Autodesk Fusion 360 part; units mm, degrees
(part 18 of 25)
  arc A5071 (10.428, 31.5912) -> (10.428, 31.9088) centre (10.428, 31.75) ccw
  arc A5072 (0.7747, 31.9088) -> (0.7747, 31.5912) centre (0.7747, 31.75) ccw
  arc A5073 (84.2253, 30.3212) -> (84.2253, 30.6388) centre (84.2253, 30.48) ccw
  arc A5074 (9.3135, 30.6388) -> (9.3135, 30.3212) centre (9.3135, 30.48) ccw
  arc A5075 (81.28, 31.2738) -> (81.28, 30.9563) centre (81.28, 31.1151) ccw
  arc A5076 (12.5375, 32.8613) -> (12.5375, 33.1788) centre (12.5375, 33.0201) ccw
  arc A5077 (0.7747, 31.2738) -> (0.7747, 30.9563) centre (0.7747, 31.1151) ccw
  arc A5078 (26.9586, 30.9563) -> (26.9586, 31.2738) centre (26.9586, 31.1151) ccw
  arc A5079 (84.2253, 29.6863) -> (84.2253, 30.0038) centre (84.2253, 29.8451) ccw
  arc A5080 (17.7173, 31.9088) -> (17.7173, 31.5912) centre (17.7173, 31.75) ccw
  arc A5081 (37.7536, 31.5912) -> (37.7536, 31.9088) centre (37.7536, 31.75) ccw
  arc A5082 (71.8947, 30.9563) -> (71.8947, 31.2738) centre (71.8947, 31.1151) ccw
  arc A5083 (66.04, 30.0038) -> (66.04, 29.6863) centre (66.04, 29.8451) ccw
  arc A5084 (67.5178, 30.6388) -> (67.5178, 30.3212) centre (67.5178, 30.48) ccw
  arc A5085 (66.04, 30.6388) -> (66.04, 30.3212) centre (66.04, 30.48) ccw
  arc A5086 (50.5114, 31.2738) -> (50.5114, 30.9563) centre (50.5114, 31.1151) ccw
  arc A5087 (49.9686, 31.5912) -> (49.9686, 31.9088) centre (49.9686, 31.75) ccw
  arc A5088 (47.9714, 33.8137) -> (47.9714, 33.4963) centre (47.9714, 33.655) ccw
  arc A5089 (1.0423, 33.4963) -> (1.0423, 33.8137) centre (1.0423, 33.655) ccw
  arc A5090 (71.8947, 32.2263) -> (71.8947, 32.5437) centre (71.8947, 32.385) ccw
  arc A5091 (67.5513, 32.5437) -> (67.5513, 32.2263) centre (67.5513, 32.385) ccw
  arc A5092 (59.1947, 32.2263) -> (59.1947, 32.5437) centre (59.1947, 32.385) ccw
  arc A5093 (4.5252, 33.1788) -> (4.5252, 32.8613) centre (4.5252, 33.0201) ccw
  arc A5094 (59.1947, 32.8613) -> (59.1947, 33.1788) centre (59.1947, 33.0201) ccw
  arc A5095 (54.786, 33.4963) -> (54.786, 33.8137) centre (54.786, 33.655) ccw
  arc A5096 (13.194, 31.9088) -> (13.194, 31.5912) centre (13.194, 31.75) ccw
  arc A5097 (56.974, 33.8137) -> (56.974, 33.4963) centre (56.974, 33.655) ccw
  arc A5098 (81.28, 32.2263) -> (81.28, 32.5437) centre (81.28, 32.385) ccw
  arc A5099 (0.7747, 33.1788) -> (0.7747, 32.8613) centre (0.7747, 33.0201) ccw
  arc A5100 (49.3336, 32.2263) -> (49.3336, 32.5437) centre (49.3336, 32.385) ccw
  arc A5101 (15.127, 31.5912) -> (15.127, 31.9088) centre (15.127, 31.75) ccw
  arc A5102 (66.04, 33.8137) -> (66.04, 33.4963) centre (66.04, 33.655) ccw
  arc A5103 (59.4491, 33.4963) -> (59.4491, 33.8137) centre (59.4491, 33.655) ccw
  arc A5104 (67.5178, 33.1788) -> (67.5178, 32.8613) centre (67.5178, 33.0201) ccw
  arc A5105 (67.2068, 33.8137) -> (67.2068, 33.4963) centre (67.2068, 33.655) ccw
  arc A5106 (72.1491, 33.4963) -> (72.1491, 33.8137) centre (72.1491, 33.655) ccw
  arc A5107 (49.2414, 32.5437) -> (49.2414, 32.2263) centre (49.2414, 32.385) ccw
  arc A5108 (1.5708, 32.8613) -> (1.5708, 33.1788) centre (1.5708, 33.0201) ccw
  arc A5109 (66.04, 32.2263) -> (66.04, 32.5437) centre (66.04, 32.385) ccw
  arc A5110 (12.559, 32.5437) -> (12.559, 32.2263) centre (12.559, 32.385) ccw
  arc A5111 (9.793, 32.2263) -> (9.793, 32.5437) centre (9.793, 32.385) ccw
  arc A5112 (81.28, 33.4963) -> (81.28, 33.8137) centre (81.28, 33.655) ccw
  arc A5113 (17.7419, 32.5437) -> (17.7419, 32.2263) centre (17.7419, 32.385) ccw
  arc A5114 (15.762, 32.2263) -> (15.762, 32.5437) centre (15.762, 32.385) ccw
  arc A5115 (66.04, 32.5437) -> (66.04, 32.2263) centre (66.04, 32.385) ccw
  arc A5116 (6.6508, 32.8613) -> (6.6508, 33.1788) centre (6.6508, 33.0201) ccw
  arc A5117 (27.6989, 33.1788) -> (27.6989, 32.8613) centre (27.6989, 33.0201) ccw
  arc A5118 (66.04, 31.9088) -> (66.04, 31.5912) centre (66.04, 31.75) ccw
  arc A5119 (49.3336, 33.4963) -> (49.3336, 33.8137) centre (49.3336, 33.655) ccw
  arc A5120 (38.3886, 32.2263) -> (38.3886, 32.5437) centre (38.3886, 32.385) ccw
  arc A5121 (52.2664, 32.5437) -> (52.2664, 32.2263) centre (52.2664, 32.385) ccw
  arc A5122 (54.9021, 32.2263) -> (54.9021, 32.5437) centre (54.9021, 32.385) ccw
  arc A5123 (71.8947, 31.5912) -> (71.8947, 31.9088) centre (71.8947, 31.75) ccw
  arc A5124 (59.1947, 31.5912) -> (59.1947, 31.9088) centre (59.1947, 31.75) ccw
  arc A5125 (49.8764, 31.9088) -> (49.8764, 31.5912) centre (49.8764, 31.75) ccw
  arc A5126 (84.2253, 31.5912) -> (84.2253, 31.9088) centre (84.2253, 31.75) ccw
  arc A5127 (56.8579, 31.9088) -> (56.8579, 31.5912) centre (56.8579, 31.75) ccw
  arc A5128 (56.8579, 32.5437) -> (56.8579, 32.2263) centre (56.8579, 32.385) ccw
  arc A5129 (81.28, 32.5437) -> (81.28, 32.2263) centre (81.28, 32.385) ccw
  arc A5130 (84.2253, 32.2263) -> (84.2253, 32.5437) centre (84.2253, 32.385) ccw
  arc A5131 (28.2956, 33.8137) -> (28.2956, 33.4963) centre (28.2956, 33.655) ccw
  arc A5132 (71.8909, 35.6205) -> (71.7694, 35.9138) centre (71.8302, 35.7672) ccw
  arc A5133 (72.6035, 1.8222) -> (72.8969, 1.9437) centre (72.7502, 1.883) ccw
  line L1815 (59.0355, 26.8859) -> (57.8045, 26.8859)
  arc A5134 (71.4301, 38.2304) -> (71.3086, 37.937) centre (71.3693, 38.0837) ccw
  line L1816 (54.0561, 37.659) -> (53.781, 37.3839)
  line L1817 (51.4155, 31.5341) -> (52.2859, 32.4045)
  arc A5135 (57.0464, 24.8968) -> (56.8218, 24.6723) centre (56.9341, 24.7846) ccw
  arc A5136 (55.0151, 36.0108) -> (55.0151, 35.6934) centre (55.0151, 35.8521) ccw
  arc A5137 (58.9232, 24.0264) -> (59.1477, 23.8018) centre (59.0355, 23.9141) ccw
  arc A5138 (72.6402, 3.234) -> (72.3227, 3.234) centre (72.4814, 3.234) ccw
  line L1818 (57.8045, 23.9141) -> (59.0355, 23.9141)
  arc A5139 (52.3982, 32.2923) -> (52.1736, 32.5168) centre (52.2859, 32.4046) ccw
  arc A5140 (72.2951, 36.0076) -> (72.0706, 36.2321) centre (72.1829, 36.1198) ccw
  arc A5141 (59.1477, 26.9982) -> (58.9232, 26.7736) centre (59.0355, 26.8859) ccw
  arc A5142 (50.0723, 31.4218) -> (50.2968, 31.6464) centre (50.1845, 31.5341) ccw
  arc A5143 (70.3249, 37.6491) -> (70.3249, 37.9666) centre (70.3249, 37.8079) ccw
  line L1819 (71.3694, 38.0837) -> (70.8706, 38.0837)
  line L1820 (72.3737, 37.0794) -> (72.1828, 37.5402)
  arc A5144 (50.1845, 34.6646) -> (50.1845, 34.3471) centre (50.1845, 34.5058) ccw
  line L1821 (72.7502, 1.8829) -> (73.2468, 1.3863)
  line L1822 (75.2467, 4.3794) -> (74.5979, 4.6482)
  line L1823 (50.1845, 34.5059) -> (49.3141, 33.6355)
  arc A5145 (53.8932, 37.2717) -> (53.6687, 37.4962) centre (53.781, 37.384) ccw
  line L1824 (71.8302, 35.7672) -> (72.1828, 36.1198)
  arc A5146 (70.8706, 35.7351) -> (70.8706, 35.4176) centre (70.8706, 35.5764) ccw
  arc A5147 (73.8956, 4.8069) -> (73.8956, 4.4894) centre (73.8956, 4.6482) ccw
  arc A5148 (57.6923, 23.8018) -> (57.9168, 24.0264) centre (57.8045, 23.9141) ccw
  arc A5149 (50.2968, 34.3936) -> (50.0723, 34.6182) centre (50.1846, 34.5059) ccw
  line L1825 (57.8045, 26.8859) -> (56.9341, 26.0155)
  arc A5150 (74.5979, 4.4894) -> (74.5979, 4.8069) centre (74.5979, 4.6482) ccw
  line L1826 (71.3694, 35.5763) -> (71.8302, 35.7672)
  arc A5151 (56.8218, 26.1277) -> (57.0464, 25.9032) centre (56.9341, 26.0155) ccw
  arc A5152 (72.8969, 3.8221) -> (72.6035, 3.9436) centre (72.7502, 3.8829) ccw
  arc A5153 (71.3694, 35.4176) -> (71.3694, 35.7351) centre (71.3694, 35.5764) ccw
  arc A5154 (52.1736, 33.2352) -> (52.3982, 33.0107) centre (52.2859, 33.123) ccw
  arc A5155 (53.6687, 37.4962) -> (53.8932, 37.2717) centre (53.781, 37.384) ccw
  arc A5156 (57.8045, 24.0729) -> (57.8045, 23.7553) centre (57.8045, 23.9141) ccw
  line L1827 (55.0151, 35.8521) -> (70.3249, 35.8521)
  arc A5157 (9.8742, 30.078) -> (9.5567, 30.078) centre (9.7155, 30.078) ccw
  arc A5158 (70.8099, 35.4296) -> (70.9314, 35.723) centre (70.8706, 35.5763) ccw
  line L1828 (52.2859, 33.1229) -> (55.0151, 35.8521)
  line L1829 (50.9029, 34.5059) -> (50.1845, 34.5059)
  arc A5159 (72.6281, 2.5925) -> (72.3348, 2.471) centre (72.4815, 2.5317) ccw
  line L1830 (72.4814, 3.234) -> (72.4814, 2.5318)
  line L1831 (70.4098, 35.7672) -> (70.8706, 35.5763)
  line L1832 (70.8706, 35.5763) -> (71.3694, 35.5763)
  arc A5160 (70.4372, 35.9644) -> (70.2126, 35.7398) centre (70.3249, 35.8521) ccw
  line L1833 (72.3737, 36.5806) -> (72.3737, 37.0794)
  arc A5161 (52.4446, 33.1229) -> (52.1271, 33.1229) centre (52.2858, 33.1229) ccw
  arc A5162 (70.3249, 35.6934) -> (70.3249, 36.0108) centre (70.3249, 35.8521) ccw
  arc A5163 (55.1273, 35.7398) -> (54.9028, 35.9644) centre (55.0151, 35.8521) ccw
  arc A5164 (50.7907, 34.6182) -> (51.0152, 34.3936) centre (50.903, 34.5059) ccw
  line L1834 (72.1828, 37.5402) -> (71.8302, 37.8928)
  arc A5165 (71.3086, 35.723) -> (71.4301, 35.4296) centre (71.3693, 35.5763) ccw
  line L1835 (52.2859, 32.4045) -> (52.2859, 33.1229)
  arc A5166 (51.3032, 31.6464) -> (51.5277, 31.4218) centre (51.4154, 31.5341) ccw
  arc A5167 (72.0706, 37.4279) -> (72.2951, 37.6524) centre (72.1829, 37.5402) ccw
  arc A5168 (59.7936, 25.9032) -> (60.0182, 26.1277) centre (59.9059, 26.0155) ccw
  arc A5169 (70.2976, 35.6549) -> (70.5221, 35.8794) centre (70.4099, 35.7672) ccw
  arc A5170 (71.7179, 35.8794) -> (71.9424, 35.6549) centre (71.8302, 35.7672) ccw
  arc A5171 (71.7694, 37.7462) -> (71.8909, 38.0395) centre (71.8302, 37.8929) ccw
  arc A5172 (71.3694, 37.9249) -> (71.3694, 38.2424) centre (71.3694, 38.0837) ccw
  arc A5173 (51.4155, 31.3754) -> (51.4155, 31.6929) centre (51.4155, 31.5342) ccw
  arc A5174 (70.5221, 37.7806) -> (70.2976, 38.0051) centre (70.4099, 37.8928) ccw
  line L1836 (73.2468, 4.3794) -> (72.7502, 3.8829)
  arc A5175 (73.359, 4.2672) -> (73.1345, 4.4917) centre (73.2468, 4.3794) ccw
  arc A5176 (82.1334, 3.7706) -> (82.3579, 3.9951) centre (82.2456, 3.8829) ccw
  arc A5177 (79.5079, 1.8522) -> (79.2834, 1.6276) centre (79.3957, 1.7399) ccw
  arc A5178 (75.7125, 1.6276) -> (75.488, 1.8522) centre (75.6003, 1.7399) ccw
  arc A5179 (49.2018, 33.7477) -> (49.4264, 33.5232) centre (49.3141, 33.6355) ccw
  arc A5180 (57.8045, 27.0446) -> (57.8045, 26.7271) centre (57.8045, 26.8859) ccw
  line L1837 (49.3141, 32.4045) -> (50.1845, 31.5341)
  arc A5181 (56.7754, 24.7845) -> (57.0928, 24.7845) centre (56.9341, 24.7845) ccw
  arc A5182 (49.4264, 32.5168) -> (49.2018, 32.2923) centre (49.3141, 32.4046) ccw
  arc A5183 (59.7471, 24.7845) -> (60.0646, 24.7845) centre (59.9059, 24.7845) ccw
  arc A5184 (72.3348, 3.2948) -> (72.6281, 3.1733) centre (72.4814, 3.234) ccw
  arc A5185 (60.0646, 26.0155) -> (59.7471, 26.0155) centre (59.9059, 26.0155) ccw
  arc A5186 (59.0355, 26.7271) -> (59.0355, 27.0446) centre (59.0355, 26.8859) ccw
  arc A5187 (60.0182, 24.6723) -> (59.7936, 24.8968) centre (59.9059, 24.7845) ccw
  arc A5188 (49.4729, 33.6355) -> (49.1554, 33.6355) centre (49.3142, 33.6355) ccw
  line L1838 (49.3141, 33.6355) -> (49.3141, 32.4045)
  line L1839 (56.9341, 24.7845) -> (57.8045, 23.9141)
  arc A5189 (50.1845, 31.6929) -> (50.1845, 31.3754) centre (50.1845, 31.5342) ccw
  line L1840 (59.9059, 24.7845) -> (59.9059, 26.0155)
  arc A5190 (72.6379, 3.9951) -> (72.8624, 3.7706) centre (72.7501, 3.8829) ccw
  arc A5191 (49.1554, 32.4045) -> (49.4729, 32.4045) centre (49.3142, 32.4045) ccw
  arc A5192 (75.3075, 1.2397) -> (75.1859, 1.533) centre (75.2467, 1.3863) ccw
  line L1841 (56.9341, 26.0155) -> (56.9341, 24.7845)
  line L1842 (73.8956, 4.6482) -> (73.2468, 4.3794)
  arc A5193 (79.6369, 1.2741) -> (79.8614, 1.4986) centre (79.7491, 1.3864) ccw
  arc A5194 (59.0355, 23.7553) -> (59.0355, 24.0729) centre (59.0355, 23.9141) ccw
  line L1843 (59.0355, 23.9141) -> (59.9059, 24.7845)
  arc A5195 (57.0928, 26.0155) -> (56.7754, 26.0155) centre (56.9341, 26.0155) ccw
  arc A5196 (75.359, 4.4917) -> (75.1344, 4.2672) centre (75.2467, 4.3794) ccw
  arc A5197 (75.488, 3.9136) -> (75.7125, 4.1382) centre (75.6003, 4.0259) ccw
  line L1844 (79.3956, 1.7399) -> (79.7492, 1.3863)
  arc A5198 (74.6586, 4.7949) -> (74.5371, 4.5015) centre (74.5978, 4.6482) ccw
  line L1845 (72.4814, 2.5318) -> (72.7502, 1.8829)
  arc A5199 (50.9029, 34.3471) -> (50.9029, 34.6646) centre (50.9029, 34.5058) ccw
  arc A5200 (57.9168, 26.7736) -> (57.6923, 26.9982) centre (57.8046, 26.8859) ccw
  arc A5201 (72.8624, 1.9952) -> (72.6379, 1.7707) centre (72.7501, 1.8829) ccw
  line L1846 (50.1845, 31.5341) -> (51.4155, 31.5341)
  arc A5202 (73.3075, 1.533) -> (73.186, 1.2397) centre (73.2468, 1.3863) ccw
  line L1847 (72.7502, 3.8829) -> (72.4814, 3.234)
  arc A5203 (72.3227, 2.5318) -> (72.6402, 2.5318) centre (72.4814, 2.5318) ccw
  arc A5204 (73.186, 4.5261) -> (73.3075, 4.2328) centre (73.2468, 4.3795) ccw
  line L1848 (59.9059, 26.0155) -> (59.0355, 26.8859)
  arc A5205 (73.8348, 0.9709) -> (73.9563, 1.2643) centre (73.8956, 1.1176) ccw
  arc A5206 (74.5371, 1.2643) -> (74.6586, 0.9709) centre (74.5978, 1.1176) ccw
  arc A5207 (75.6003, 1.8986) -> (75.6003, 1.5812) centre (75.6003, 1.7399) ccw
  arc A5208 (82.3678, 3.1733) -> (82.6611, 3.2948) centre (82.5145, 3.2341) ccw
  arc A5209 (79.8614, 4.2672) -> (79.6369, 4.4917) centre (79.7491, 4.3794) ccw
  arc A5210 (81.0395, 1.2643) -> (81.161, 0.9709) centre (81.1003, 1.1176) ccw
  arc A5211 (75.1859, 4.2328) -> (75.3075, 4.5261) centre (75.2467, 4.3794) ccw
  arc A5212 (6.75, 12.0328) -> (6.4325, 12.0328) centre (6.5913, 12.0328) ccw
  arc A5213 (6.4325, 10.8018) -> (6.75, 10.8018) centre (6.5913, 10.8018) ccw
  arc A5214 (73.9563, 4.5015) -> (73.8348, 4.7949) centre (73.8956, 4.6482) ccw
  line L1849 (75.6003, 4.0259) -> (75.2467, 4.3794)
  arc A5215 (74.5979, 0.9589) -> (74.5979, 1.2764) centre (74.5979, 1.1177) ccw
  arc A5216 (82.099, 1.9437) -> (82.3924, 1.8222) centre (82.2457, 1.883) ccw
  arc A5217 (73.1345, 1.2741) -> (73.359, 1.4986) centre (73.2468, 1.3864) ccw
  arc A5218 (79.3956, 3.8671) -> (79.3956, 4.1846) centre (79.3956, 4.0259) ccw
  line L1850 (6.5913, 10.8018) -> (6.5913, 12.0328)
  arc A5219 (82.6732, 3.234) -> (82.3557, 3.234) centre (82.5145, 3.234) ccw
  line L1851 (80.398, 1.1176) -> (81.1003, 1.1176)
  arc A5220 (73.8956, 1.2764) -> (73.8956, 0.9589) centre (73.8956, 1.1177) ccw
  line L1852 (74.5979, 4.6482) -> (73.8956, 4.6482)
  line L1853 (74.5979, 1.1176) -> (75.2467, 1.3863)
  arc A5221 (79.3956, 1.5812) -> (79.3956, 1.8986) centre (79.3956, 1.7399) ccw
  arc A5222 (3.7318, 10.9141) -> (3.5072, 10.6896) centre (3.6195, 10.8018) ccw
  arc A5223 (82.3924, 3.9436) -> (82.099, 3.8221) centre (82.2457, 3.8829) ccw
  line L1854 (82.5144, 2.5318) -> (82.5144, 3.234)
  line L1855 (3.6576, 3.7973) -> (3.6576, 3.2134)
  arc A5224 (5.0673, 2.2288) -> (5.0673, 2.5463) centre (5.0673, 2.3876) ccw
  line L1856 (82.5144, 3.234) -> (82.2457, 3.8829)
  line L1857 (73.8956, 1.1176) -> (74.5979, 1.1176)
  arc A5225 (80.3372, 0.9709) -> (80.4587, 1.2643) centre (80.398, 1.1176) ccw
  arc A5226 (80.398, 1.2764) -> (80.398, 0.9589) centre (80.398, 1.1177) ccw
  line L1858 (81.1003, 1.1176) -> (81.7491, 1.3863)
  arc A5227 (81.161, 4.7949) -> (81.0395, 4.5015) centre (81.1003, 4.6482) ccw
  line L1859 (79.3956, 4.0259) -> (75.6003, 4.0259)
  line L1860 (81.1003, 4.6482) -> (80.398, 4.6482)
  arc A5228 (6.5893, 3.1011) -> (6.3647, 3.3256) centre (6.477, 3.2134) ccw
  line L1861 (5.6512, 2.3876) -> (6.477, 3.2134)
  arc A5229 (82.6611, 2.471) -> (82.3678, 2.5925) centre (82.5145, 2.5318) ccw
  arc A5230 (5.0673, 2.5463) -> (5.0673, 2.2288) centre (5.0673, 2.3876) ccw
  line L1862 (3.6195, 12.0328) -> (3.6195, 10.8018)
  line L1863 (75.6003, 1.7399) -> (79.3956, 1.7399)
  line L1864 (4.4834, 2.3876) -> (5.0673, 2.3876)
  arc A5231 (4.4899, 13.0619) -> (4.4899, 12.7444) centre (4.4899, 12.9032) ccw
  line L1865 (3.6195, 10.8018) -> (4.1275, 10.2938)
  line L1866 (80.398, 4.6482) -> (79.7492, 4.3794)
  line L1867 (82.2457, 3.8829) -> (81.7491, 4.3794)
  line L1868 (81.7491, 4.3794) -> (81.1003, 4.6482)
  line L1869 (81.7491, 1.3863) -> (82.2457, 1.8829)
  arc A5232 (79.2834, 4.1382) -> (79.5079, 3.9136) centre (79.3957, 4.0259) ccw
  arc A5233 (4.9086, 2.3876) -> (5.2261, 2.3876) centre (5.0674, 2.3876) ccw
  arc A5234 (5.6512, 2.2288) -> (5.6512, 2.5463) centre (5.6512, 2.3876) ccw
  arc A5235 (81.6368, 1.4986) -> (81.8614, 1.2741) centre (81.7491, 1.3864) ccw
  line L1870 (4.1275, 7.7503) -> (3.4036, 7.0264)
  arc A5236 (5.539, 2.4999) -> (5.7635, 2.2753) centre (5.6513, 2.3876) ccw
  line L1871 (3.4036, 7.0264) -> (3.4036, 5.6482)
  arc A5237 (4.0518, 4.7754) -> (4.2763, 4.9999) centre (4.1641, 4.8877) ccw
  arc A5238 (5.0673, 3.6386) -> (5.0673, 3.9561) centre (5.0673, 3.7973) ccw
  arc A5239 (81.1003, 0.9589) -> (81.1003, 1.2764) centre (81.1003, 1.1177) ccw
  line L1872 (5.0673, 2.3876) -> (5.6512, 2.3876)
  arc A5240 (5.226, 3.7973) -> (4.9085, 3.7973) centre (5.0672, 3.7973) ccw
  arc A5241 (81.1003, 4.4894) -> (81.1003, 4.8069) centre (81.1003, 4.6482) ccw
  arc A5242 (80.4587, 4.5015) -> (80.3372, 4.7949) centre (80.398, 4.6482) ccw
  line L1873 (82.2457, 1.8829) -> (82.5144, 2.5318)
  line L1874 (5.7209, 12.9032) -> (4.4899, 12.9032)
  arc A5243 (3.5072, 12.145) -> (3.7318, 11.9205) centre (3.6195, 12.0328) ccw
  arc A5244 (5.2261, 3.7973) -> (4.9086, 3.7973) centre (5.0674, 3.7973) ccw
  line L1875 (73.2468, 1.3863) -> (73.8956, 1.1176)
  arc A5245 (81.6883, 4.2328) -> (81.8099, 4.5261) centre (81.7491, 4.3794) ccw
  arc A5246 (4.2863, 10.2938) -> (3.9688, 10.2938) centre (4.1276, 10.2938) ccw
  arc A5247 (79.6884, 4.5261) -> (79.8099, 4.2328) centre (79.7492, 4.3795) ccw
  arc A5248 (6.479, 11.9205) -> (6.7036, 12.145) centre (6.5913, 12.0328) ccw
  arc A5249 (3.6576, 3.9561) -> (3.6576, 3.6386) centre (3.6576, 3.7973) ccw
  arc A5250 (3.5623, 7.0264) -> (3.2449, 7.0264) centre (3.4036, 7.0264) ccw
  arc A5251 (80.398, 4.8069) -> (80.398, 4.4894) centre (80.398, 4.6482) ccw
  arc A5252 (81.8099, 1.2397) -> (81.6883, 1.533) centre (81.7491, 1.3864) ccw
  line L1876 (75.2467, 1.3863) -> (75.6003, 1.7399)
  arc A5253 (75.1344, 1.4986) -> (75.359, 1.2741) centre (75.2467, 1.3863) ccw
  arc A5254 (79.8099, 1.533) -> (79.6884, 1.2397) centre (79.7492, 1.3863) ccw
  line L1877 (79.7492, 4.3794) -> (79.3956, 4.0259)
  line L1878 (79.7492, 1.3863) -> (80.398, 1.1176)
  arc A5255 (4.2763, 4.7754) -> (4.0518, 4.9999) centre (4.1641, 4.8877) ccw
  arc A5256 (82.3557, 2.5318) -> (82.6732, 2.5318) centre (82.5145, 2.5318) ccw
  arc A5257 (81.8614, 4.4917) -> (81.6368, 4.2672) centre (81.7491, 4.3794) ccw
  arc A5258 (82.3579, 1.7707) -> (82.1334, 1.9952) centre (82.2456, 1.8829) ccw
  arc A5259 (75.6003, 4.1846) -> (75.6003, 3.8671) centre (75.6003, 4.0259) ccw
  arc A5260 (6.5722, 5.6482) -> (6.8897, 5.6482) centre (6.731, 5.6482) ccw
  arc A5261 (5.971, 10.4061) -> (6.1956, 10.1816) centre (6.0833, 10.2938) ccw
  arc A5262 (83.5257, 20.3759) -> (83.2324, 20.2544) centre (83.379, 20.3152) ccw
  arc A5263 (82.9917, 14.9042) -> (83.2162, 14.6797) centre (83.1039, 14.792) ccw
  line L1879 (5.0673, 3.7973) -> (5.0673, 2.3876)
  arc A5264 (3.9688, 7.7503) -> (4.2863, 7.7503) centre (4.1276, 7.7503) ccw
  arc A5265 (4.0152, 10.1816) -> (4.2398, 10.4061) centre (4.1275, 10.2938) ccw
  arc A5266 (3.5453, 4.4935) -> (3.7699, 4.269) centre (3.6576, 4.3813) ccw
  arc A5267 (3.7783, 12.0328) -> (3.4608, 12.0328) centre (3.6196, 12.0328) ccw
  line L1880 (6.477, 3.2134) -> (6.477, 3.7973)
  line L1881 (84.1629, 11.8305) -> (84.1629, 13.0615)
  arc A5268 (83.2925, 13.7731) -> (83.2925, 14.0906) centre (83.2925, 13.9319) ccw
  arc A5269 (3.4608, 10.8018) -> (3.7783, 10.8018) centre (3.6196, 10.8018) ccw
  arc A5270 (83.3812, 19.895) -> (83.6746, 20.0165) centre (83.5279, 19.9558) ccw
  line L1882 (5.0673, 3.7973) -> (6.477, 3.7973)
  arc A5271 (3.2449, 5.6482) -> (3.5623, 5.6482) centre (3.4036, 5.6482) ccw
  line L1883 (83.5279, 19.9557) -> (83.379, 20.3151)
  arc A5272 (4.4834, 2.5463) -> (4.4834, 2.2289) centre (4.4834, 2.3876) ccw
  arc A5273 (3.7699, 3.3256) -> (3.5453, 3.1011) centre (3.6576, 3.2134) ccw
  arc A5274 (6.0828, 4.9999) -> (5.8583, 4.7754) centre (5.9706, 4.8877) ccw
  line L1884 (83.379, 20.3151) -> (82.4865, 21.2077)
  arc A5275 (82.5987, 21.3199) -> (82.3742, 21.0954) centre (82.4864, 21.2077) ccw
  line L1885 (84.1629, 13.0615) -> (83.2925, 13.9319)
  arc A5276 (83.2668, 20.2029) -> (83.4913, 20.4274) centre (83.3791, 20.3151) ccw
  arc A5277 (4.9086, 3.7973) -> (5.2261, 3.7973) centre (5.0674, 3.7973) ccw
  arc A5278 (6.7036, 10.6896) -> (6.479, 10.9141) centre (6.5913, 10.8019) ccw
  arc A5279 (4.9085, 3.7973) -> (5.226, 3.7973) centre (5.0672, 3.7973) ccw
  line L1886 (4.1641, 4.8877) -> (3.6576, 4.3812)
  arc A5280 (83.6866, 19.9557) -> (83.3691, 19.9557) centre (83.5279, 19.9557) ccw
  line L1887 (83.1039, 14.792) -> (83.379, 15.0671)
  arc A5281 (6.6357, 4.3812) -> (6.3182, 4.3812) centre (6.477, 4.3812) ccw
  arc A5282 (4.2398, 7.6381) -> (4.0152, 7.8626) centre (4.1275, 7.7503) ccw
  line L1888 (82.4865, 21.2077) -> (82.4865, 21.4135)
  line L1889 (3.6576, 3.2134) -> (4.4834, 2.3876)
  line L1890 (6.5913, 12.0328) -> (5.7209, 12.9032)
  arc A5283 (4.9085, 2.3876) -> (5.226, 2.3876) centre (5.0672, 2.3876) ccw
  arc A5284 (3.8163, 3.7973) -> (3.4989, 3.7973) centre (3.6576, 3.7973) ccw
  arc A5285 (5.0673, 3.6385) -> (5.0673, 3.956) centre (5.0673, 3.7973) ccw
  arc A5286 (83.4047, 14.0442) -> (83.1802, 13.8196) centre (83.2924, 13.9319) ccw
  arc A5287 (3.5159, 5.7604) -> (3.2913, 5.5359) centre (3.4036, 5.6481) ccw
  arc A5288 (4.6022, 12.7909) -> (4.3777, 13.0155) centre (4.4899, 12.9032) ccw
  line L1891 (3.6576, 4.3812) -> (3.6576, 3.7973)
  arc A5289 (5.0673, 3.956) -> (5.0673, 3.6385) centre (5.0673, 3.7973) ccw
  arc A5290 (6.6357, 3.7973) -> (6.3182, 3.7973) centre (6.477, 3.7973) ccw
  arc A5291 (5.226, 3.7973) -> (4.9085, 3.7973) centre (5.0672, 3.7973) ccw
  arc A5292 (5.9245, 7.6741) -> (6.242, 7.6741) centre (6.0833, 7.6741) ccw
  line L1892 (3.6576, 3.7973) -> (5.0673, 3.7973)
  line L1893 (5.0673, 2.3876) -> (5.0673, 3.7973)
  arc A5293 (5.7209, 12.7444) -> (5.7209, 13.0619) centre (5.7209, 12.9032) ccw
  line L1894 (3.4036, 5.6482) -> (4.1641, 4.8877)
  arc A5294 (3.6576, 3.956) -> (3.6576, 3.6385) centre (3.6576, 3.7973) ccw
  arc A5295 (3.2913, 7.1387) -> (3.5159, 6.9142) centre (3.4036, 7.0265) ccw
  line L1895 (4.1275, 10.2938) -> (4.1275, 7.7503)
  arc A5296 (4.3711, 2.2753) -> (4.5956, 2.4999) centre (4.4834, 2.3876) ccw
  line L1896 (4.4899, 12.9032) -> (3.6195, 12.0328)
  arc A5297 (5.0673, 3.956) -> (5.0673, 3.6385) centre (5.0673, 3.7973) ccw
  arc A5298 (3.4989, 3.2134) -> (3.8163, 3.2134) centre (3.6576, 3.2134) ccw
  arc A5299 (83.6746, 15.3657) -> (83.3812, 15.4872) centre (83.5279, 15.4265) ccw
  arc A5300 (3.8163, 4.3812) -> (3.4989, 4.3812) centre (3.6576, 4.3812) ccw
  line L1897 (5.0673, 3.7973) -> (3.6576, 3.7973)
  arc A5301 (5.0673, 3.6385) -> (5.0673, 3.956) centre (5.0673, 3.7973) ccw
  arc A5302 (3.4989, 3.7973) -> (3.8163, 3.7973) centre (3.6576, 3.7973) ccw
  arc A5303 (83.3691, 15.4265) -> (83.6866, 15.4265) centre (83.5279, 15.4265) ccw
  arc A5304 (5.8331, 13.0155) -> (5.6086, 12.7909) centre (5.7208, 12.9032) ccw
  arc A5305 (6.3182, 3.7973) -> (6.6357, 3.7973) centre (6.477, 3.7973) ccw
  line L1898 (81.0723, 23.0759) -> (80.3701, 23.0759)
  arc A5306 (75.6031, 22.1983) -> (75.8276, 22.4228) centre (75.7154, 22.3105) ccw
  line L1899 (83.1039, 22.031) -> (83.379, 22.3061)
  line L1900 (83.379, 15.0671) -> (83.5279, 15.4265)
  line L1901 (75.2188, 22.8071) -> (74.5699, 23.0759)
  arc A5307 (74.6307, 23.2226) -> (74.5092, 22.9292) centre (74.57, 23.0759) ccw
  line L1902 (83.1655, 26.8859) -> (81.9345, 26.8859)
  line L1903 (81.0641, 26.0155) -> (81.0641, 24.7845)
  arc A5308 (82.2439, 14.0906) -> (82.2439, 13.7731) centre (82.2439, 13.9319) ccw
  line L1904 (84.0359, 24.7845) -> (84.0359, 26.0155)
  arc A5309 (82.0468, 26.7736) -> (81.8223, 26.9982) centre (81.9346, 26.8859) ccw
  line L1905 (6.0833, 7.6741) -> (6.0833, 10.2938)
  line L1906 (75.7153, 22.3106) -> (75.2188, 22.8071)
  arc A5310 (6.8897, 7.0264) -> (6.5722, 7.0264) centre (6.731, 7.0264) ccw
  arc A5311 (82.3277, 21.2077) -> (82.6452, 21.2077) centre (82.4864, 21.2077) ccw
  arc A5312 (6.477, 3.6386) -> (6.477, 3.9561) centre (6.477, 3.7973) ccw
  line L1907 (83.2925, 13.9319) -> (82.2439, 13.9319)
  arc A5313 (84.1946, 26.0155) -> (83.8771, 26.0155) centre (84.0358, 26.0155) ccw
  arc A5314 (81.1797, 23.0972) -> (81.4042, 22.8727) centre (81.2919, 22.9849) ccw
  arc A5315 (80.4308, 22.9292) -> (80.3093, 23.2226) centre (80.3701, 23.0759) ccw
  arc A5316 (79.2155, 22.1297) -> (79.2155, 22.4472) centre (79.2155, 22.2885) ccw
  arc A5317 (82.1316, 14.0442) -> (82.3561, 13.8196) centre (82.2439, 13.9319) ccw
  line L1908 (83.5279, 15.4265) -> (83.5279, 19.9557)
  arc A5318 (83.6746, 22.6047) -> (83.3812, 22.7262) centre (83.5279, 22.6654) ccw
  line L1909 (83.5279, 24.2765) -> (84.0359, 24.7845)
  arc A5319 (81.1331, 23.2226) -> (81.0116, 22.9292) centre (81.0724, 23.0759) ccw
  arc A5320 (81.2312, 22.8383) -> (81.3527, 23.1316) centre (81.2919, 22.985) ccw
  arc A5321 (84.3216, 13.0615) -> (84.0041, 13.0615) centre (84.1629, 13.0615) ccw
  arc A5322 (6.242, 10.2938) -> (5.9245, 10.2938) centre (6.0833, 10.2938) ccw
  line L1910 (6.477, 4.3812) -> (5.9705, 4.8877)
  arc A5323 (79.1124, 22.4228) -> (79.3369, 22.1983) centre (79.2246, 22.3105) ccw
  arc A5324 (79.8335, 22.6949) -> (79.609, 22.9194) centre (79.7212, 22.8072) ccw
  arc A5325 (83.6866, 24.2765) -> (83.3691, 24.2765) centre (83.5279, 24.2765) ccw
  line L1911 (6.477, 3.7973) -> (5.0673, 3.7973)
  line L1912 (6.477, 3.7973) -> (6.477, 4.3812)
  line L1913 (79.2246, 22.3106) -> (79.2155, 22.2885)
  arc A5326 (84.0506, 12.9492) -> (84.2752, 13.1737) centre (84.1629, 13.0615) ccw
  line L1914 (6.0833, 10.2938) -> (6.5913, 10.8018)
  arc A5327 (6.1955, 7.7864) -> (5.971, 7.5619) centre (6.0832, 7.6742) ccw
  line L1915 (82.2439, 13.9319) -> (83.1039, 14.792)
  arc A5328 (6.3647, 4.269) -> (6.5893, 4.4935) centre (6.477, 4.3813) ccw
  arc A5329 (83.4913, 14.9548) -> (83.2668, 15.1793) centre (83.3791, 15.0671) ccw
  arc A5330 (84.0041, 11.8305) -> (84.3216, 11.8305) centre (84.1629, 11.8305) ccw
  arc A5331 (5.2261, 3.7973) -> (4.9086, 3.7973) centre (5.0674, 3.7973) ccw
  arc A5332 (83.2324, 15.1278) -> (83.5257, 15.0063) centre (83.3791, 15.0671) ccw
  line L1916 (5.9705, 4.8877) -> (6.731, 5.6482)
  arc A5333 (5.0673, 3.9561) -> (5.0673, 3.6386) centre (5.0673, 3.7973) ccw
  arc A5334 (6.6187, 6.9142) -> (6.8432, 7.1387) centre (6.7309, 7.0264) ccw
  line L1917 (82.4865, 21.4135) -> (83.1039, 22.031)
  line L1918 (79.2155, 22.2885) -> (75.7245, 22.2885)
  arc A5335 (83.2162, 21.9187) -> (82.9917, 22.1432) centre (83.1039, 22.0309) ccw
  arc A5336 (83.2162, 14.6797) -> (82.9917, 14.9042) centre (83.1039, 14.7919) ccw
  line L1919 (6.731, 5.6482) -> (6.731, 7.0264)
  arc A5337 (6.8432, 5.5359) -> (6.6187, 5.7604) centre (6.7309, 5.6482) ccw
  arc A5338 (6.3182, 3.2134) -> (6.6357, 3.2134) centre (6.477, 3.2134) ccw
  arc A5339 (82.6452, 21.4135) -> (82.3277, 21.4135) centre (82.4864, 21.4135) ccw
  arc A5340 (6.477, 3.6385) -> (6.477, 3.956) centre (6.477, 3.7973) ccw
  arc A5341 (5.8583, 4.9999) -> (6.0828, 4.7754) centre (5.9706, 4.8877) ccw
  line L1920 (6.731, 7.0264) -> (6.0833, 7.6741)
  arc A5342 (75.7245, 22.4472) -> (75.7245, 22.1297) centre (75.7245, 22.2885) ccw
  arc A5343 (81.9345, 27.0446) -> (81.9345, 26.7271) centre (81.9345, 26.8859) ccw
  line L1921 (81.5721, 24.2765) -> (81.5721, 23.2651)
  arc A5344 (79.3713, 22.2498) -> (79.078, 22.3713) centre (79.2247, 22.3105) ccw
  arc A5345 (81.1331, 18.7014) -> (81.0116, 18.408) centre (81.0724, 18.5547) ccw
  arc A5346 (81.4042, 19.7485) -> (81.1797, 19.524) centre (81.2919, 19.6363) ccw
  arc A5347 (81.1764, 24.8968) -> (80.9518, 24.6723) centre (81.0641, 24.7846) ccw
  line L1922 (81.5721, 23.2651) -> (81.292, 22.9849)
  arc A5348 (83.8771, 24.7845) -> (84.1946, 24.7845) centre (84.0358, 24.7845) ccw
  arc A5349 (75.158, 22.6605) -> (75.2795, 22.9538) centre (75.2188, 22.8072) ccw
  line L1923 (83.379, 22.3061) -> (83.5279, 22.6655)
  arc A5350 (83.3691, 22.6655) -> (83.6866, 22.6655) centre (83.5279, 22.6655) ccw
  line L1924 (74.5699, 23.0759) -> (73.8677, 23.0759)
  arc A5351 (72.5756, 20.2499) -> (72.8689, 20.3714) centre (72.7223, 20.3107) ccw
  arc A5352 (74.5092, 19.692) -> (74.6307, 19.3986) centre (74.57, 19.5453) ccw
  arc A5353 (80.3093, 19.3986) -> (80.4308, 19.692) centre (80.3701, 19.5453) ccw
  arc A5354 (81.4598, 24.1643) -> (81.6844, 24.3888) centre (81.5721, 24.2766) ccw
  arc A5355 (79.2155, 20.174) -> (79.2155, 20.4915) centre (79.2155, 20.3328) ccw
  line L1925 (81.0723, 18.5547) -> (80.3701, 18.5547)
  line L1926 (72.7223, 22.3106) -> (72.4535, 21.6617)
  arc A5356 (73.2796, 19.9607) -> (73.1581, 19.6674) centre (73.2189, 19.8141) ccw
  arc A5357 (80.9518, 26.1277) -> (81.1764, 25.9032) centre (81.0641, 26.0155) ccw
  arc A5358 (83.4913, 22.1938) -> (83.2668, 22.4183) centre (83.3791, 22.306) ccw
  arc A5359 (75.1065, 19.9263) -> (75.331, 19.7018) centre (75.2188, 19.814) ccw
  arc A5360 (74.5699, 19.3865) -> (74.5699, 19.7041) centre (74.5699, 19.5453) ccw
  arc A5361 (72.3068, 21.7225) -> (72.6002, 21.601) centre (72.4535, 21.6617) ccw
  arc A5362 (79.078, 20.2499) -> (79.3713, 20.3714) centre (79.2247, 20.3107) ccw
  line L1927 (79.2246, 20.3106) -> (79.7212, 19.8141)
  arc A5363 (81.5113, 18.201) -> (81.6329, 18.4944) centre (81.5721, 18.3477) ccw
  line L1928 (79.7212, 19.8141) -> (80.3701, 19.5453)
  arc A5364 (81.4134, 23.2651) -> (81.7309, 23.2651) centre (81.5722, 23.2651) ccw
  arc A5365 (83.9236, 25.9032) -> (84.1482, 26.1277) centre (84.0359, 26.0154) ccw
  line L1929 (72.4535, 21.6617) -> (72.4535, 20.9595)
  arc A5366 (72.61, 22.4228) -> (72.8345, 22.1983) centre (72.7223, 22.3105) ccw
  arc A5367 (72.2948, 20.9595) -> (72.6123, 20.9595) centre (72.4536, 20.9595) ccw
  arc A5368 (82.3742, 21.5258) -> (82.5987, 21.3013) centre (82.4864, 21.4136) ccw
  arc A5369 (81.0723, 19.3865) -> (81.0723, 19.7041) centre (81.0723, 19.5453) ccw
  line L1930 (81.292, 22.9849) -> (81.0723, 23.0759)
  arc A5370 (81.2229, 26.0155) -> (80.9054, 26.0155) centre (81.0641, 26.0155) ccw
  arc A5371 (84.1481, 24.6723) -> (83.9236, 24.8968) centre (84.0358, 24.7845) ccw
  line L1931 (84.0359, 26.0155) -> (83.1655, 26.8859)
  arc A5372 (83.4156, 24.3888) -> (83.6401, 24.1643) centre (83.5279, 24.2766) ccw
  line L1932 (81.9345, 26.8859) -> (81.0641, 26.0155)
  arc A5373 (80.9054, 24.7845) -> (81.2229, 24.7845) centre (81.0641, 24.7845) ccw
  line L1933 (73.8677, 23.0759) -> (73.2188, 22.8071)
  line L1934 (83.5279, 22.6655) -> (83.5279, 24.2765)
  line L1935 (72.7223, 20.3106) -> (73.2188, 19.8141)
  arc A5374 (79.782, 19.9607) -> (79.6605, 19.6674) centre (79.7212, 19.8141) ccw
  line L1936 (79.7212, 22.8071) -> (79.2246, 22.3106)
  line L1937 (75.7153, 20.3106) -> (75.7245, 20.3327)
  arc A5375 (75.862, 22.3713) -> (75.5687, 22.2498) centre (75.7154, 22.3105) ccw
  line L1938 (80.3701, 23.0759) -> (79.7212, 22.8071)
  arc A5376 (83.2324, 22.3668) -> (83.5257, 22.2453) centre (83.3791, 22.3061) ccw
  arc A5377 (75.331, 22.9194) -> (75.1065, 22.6949) centre (75.2188, 22.8072) ccw
  arc A5378 (75.5778, 22.2278) -> (75.8712, 22.3492) centre (75.7245, 22.2885) ccw
  line L1939 (81.0641, 24.7845) -> (81.5721, 24.2765)
  arc A5379 (83.2777, 26.9982) -> (83.0532, 26.7736) centre (83.1655, 26.8859) ccw
  arc A5380 (81.0723, 22.9171) -> (81.0723, 23.2346) centre (81.0723, 23.0758) ccw
  arc A5381 (79.6605, 22.9538) -> (79.782, 22.6605) centre (79.7212, 22.8072) ccw
  arc A5382 (83.1655, 26.7271) -> (83.1655, 27.0446) centre (83.1655, 26.8859) ccw
  arc A5383 (80.3701, 23.2346) -> (80.3701, 22.9171) centre (80.3701, 23.0758) ccw
  arc A5384 (81.6844, 23.1528) -> (81.4598, 23.3773) centre (81.5721, 23.2651) ccw
  arc A5385 (81.7309, 24.2765) -> (81.4134, 24.2765) centre (81.5722, 24.2765) ccw
  arc A5386 (82.9917, 22.1432) -> (83.2162, 21.9187) centre (83.1039, 22.031) ccw
  line L1940 (75.7245, 22.2885) -> (75.7153, 22.3106)
  arc A5387 (79.0688, 22.3492) -> (79.3622, 22.2278) centre (79.2155, 22.2885) ccw
  arc A5388 (81.4598, 19.2439) -> (81.6844, 19.4684) centre (81.5721, 19.3562) ccw
  line L1941 (72.4535, 20.9595) -> (72.7223, 20.3106)
  arc A5389 (72.39, 24.0093) -> (72.39, 24.3268) centre (72.39, 24.1681) ccw
  arc A5390 (71.8797, 24.3268) -> (71.8797, 24.0094) centre (71.8797, 24.1681) ccw
  arc A5391 (72.2313, 24.1681) -> (72.5488, 24.1681) centre (72.3901, 24.1681) ccw
  line L1942 (73.8677, 19.5453) -> (74.5699, 19.5453)
  arc A5392 (72.39, 25.2412) -> (72.39, 25.5587) centre (72.39, 25.4) ccw
  line L1943 (81.5721, 19.3561) -> (81.5721, 18.3477)
  arc A5393 (80.3701, 19.7041) -> (80.3701, 19.3865) centre (80.3701, 19.5453) ccw
  arc A5394 (79.3369, 20.4229) -> (79.1124, 20.1984) centre (79.2247, 20.3106) ccw
  arc A5395 (73.8677, 19.7041) -> (73.8677, 19.3865) centre (73.8677, 19.5453) ccw
  arc A5396 (73.3311, 18.1737) -> (73.1066, 18.3982) centre (73.2189, 18.2859) ccw
  arc A5397 (72.5487, 25.4) -> (72.2312, 25.4) centre (72.3899, 25.4) ccw
  line L1944 (69.8039, 19.4425) -> (70.0659, 19.7045)
  arc A5398 (73.1066, 19.7018) -> (73.3311, 19.9263) centre (73.2189, 19.8141) ccw
  arc A5399 (71.7675, 24.0558) -> (71.992, 24.2804) centre (71.8798, 24.1681) ccw
  line L1945 (73.2188, 22.8071) -> (72.7223, 22.3106)
  line L1946 (80.3701, 19.5453) -> (81.0723, 19.5453)
  arc A5400 (72.8653, 17.7736) -> (72.8653, 18.0911) centre (72.8653, 17.9323) ccw
  arc A5401 (81.4134, 18.3477) -> (81.7309, 18.3477) centre (81.5722, 18.3477) ccw
  arc A5402 (79.609, 19.7018) -> (79.8335, 19.9263) centre (79.7212, 19.8141) ccw
  arc A5403 (74.6307, 18.7014) -> (74.5092, 18.408) centre (74.57, 18.5547) ccw
  line L1947 (70.0659, 19.7045) -> (70.0659, 20.1895)
  line L1948 (80.3701, 18.5547) -> (79.7212, 18.2859)
  line L1949 (74.5699, 18.5547) -> (73.8677, 18.5547)
  arc A5404 (69.9071, 19.7045) -> (70.2246, 19.7045) centre (70.0658, 19.7045) ccw
  arc A5405 (81.3527, 19.4896) -> (81.2312, 19.7829) centre (81.292, 19.6363) ccw
  line L1950 (79.3677, 17.9324) -> (75.5723, 17.9324)
  arc A5406 (72.8689, 22.2498) -> (72.5756, 22.3713) centre (72.7223, 22.3105) ccw
  line L1951 (75.7245, 20.3327) -> (79.2155, 20.3327)
  arc A5407 (71.7403, 24.5321) -> (71.5157, 24.3076) centre (71.628, 24.4198) ccw
  line L1952 (73.2188, 18.2859) -> (72.8653, 17.9324)
  arc A5408 (75.331, 18.3982) -> (75.1065, 18.1737) centre (75.2188, 18.2859) ccw
  arc A5409 (75.8276, 20.1984) -> (75.6031, 20.4229) centre (75.7154, 20.3106) ccw
  line L1953 (72.39, 25.4) -> (72.39, 24.1681)
  arc A5410 (73.8069, 19.3986) -> (73.9284, 19.692) centre (73.8676, 19.5453) ccw
  arc A5411 (75.2795, 19.6674) -> (75.158, 19.9607) centre (75.2188, 19.8141) ccw
  arc A5412 (72.6002, 21.0202) -> (72.3068, 20.8987) centre (72.4535, 20.9595) ccw
  arc A5413 (79.3622, 20.3934) -> (79.0688, 20.272) centre (79.2155, 20.3327) ccw
  arc A5414 (81.7309, 19.3561) -> (81.4134, 19.3561) centre (81.5722, 19.3561) ccw
  line L1954 (71.628, 24.4198) -> (71.8797, 24.1681)
  line L1955 (75.2188, 19.8141) -> (75.7153, 20.3106)
  arc A5415 (73.1581, 22.9538) -> (73.2796, 22.6605) centre (73.2189, 22.8072) ccw
  arc A5416 (72.39, 25.5587) -> (72.39, 25.2412) centre (72.39, 25.4) ccw
  arc A5417 (72.5488, 25.4) -> (72.2313, 25.4) centre (72.3901, 25.4) ccw
  arc A5418 (81.0723, 18.3959) -> (81.0723, 18.7134) centre (81.0723, 18.5547) ccw
  line L1956 (73.2188, 19.8141) -> (73.8677, 19.5453)
  line L1957 (73.8677, 18.5547) -> (73.2188, 18.2859)
  line L1958 (81.292, 19.6363) -> (81.5721, 19.3561)
  arc A5419 (72.8345, 20.4229) -> (72.61, 20.1984) centre (72.7223, 20.3106) ccw
  line L1959 (81.5721, 18.3477) -> (81.0723, 18.5547)
  arc A5420 (75.7245, 20.4915) -> (75.7245, 20.174) centre (75.7245, 20.3328) ccw
  arc A5421 (73.9284, 22.9292) -> (73.8069, 23.2226) centre (73.8676, 23.0759) ccw
  line L1960 (79.2155, 20.3327) -> (79.2246, 20.3106)
  line L1961 (74.5699, 19.5453) -> (75.2188, 19.8141)
  arc A5422 (73.3311, 22.6949) -> (73.1066, 22.9194) centre (73.2189, 22.8072) ccw
  arc A5423 (73.8677, 23.2346) -> (73.8677, 22.9171) centre (73.8677, 23.0758) ccw
  arc A5424 (71.3073, 21.6383) -> (71.6007, 21.5168) centre (71.454, 21.5776) ccw
  arc A5425 (75.5687, 20.3714) -> (75.862, 20.2499) centre (75.7154, 20.3106) ccw
  line L1962 (71.628, 21.9976) -> (71.628, 24.4198)
  arc A5426 (81.0116, 19.692) -> (81.1331, 19.3986) centre (81.0724, 19.5453) ccw
  arc A5427 (72.6123, 21.6617) -> (72.2948, 21.6617) centre (72.4536, 21.6617) ccw
  arc A5428 (74.5699, 22.9171) -> (74.5699, 23.2346) centre (74.5699, 23.0758) ccw
  line L1963 (81.0723, 19.5453) -> (81.292, 19.6363)
  arc A5429 (73.1581, 18.4326) -> (73.2796, 18.1393) centre (73.2189, 18.2859) ccw
  arc A5430 (75.8712, 20.272) -> (75.5778, 20.3934) centre (75.7245, 20.3327) ccw
  arc A5431 (72.39, 25.2413) -> (72.39, 25.5588) centre (72.39, 25.4001) ccw
  arc A5432 (73.0125, 26.7442) -> (72.788, 26.5196) centre (72.9002, 26.6319) ccw
  arc A5433 (74.9617, 29.4567) -> (74.6442, 29.4567) centre (74.8029, 29.4567) ccw
  line L1964 (71.8797, 24.1681) -> (72.39, 24.1681)
  arc A5434 (71.7747, 21.9369) -> (71.4813, 22.0584) centre (71.628, 21.9977) ccw
  arc A5435 (72.2312, 24.1681) -> (72.5487, 24.1681) centre (72.3899, 24.1681) ccw
  arc A5436 (73.7806, 25.9103) -> (73.4631, 25.9103) centre (73.6218, 25.9103) ccw
  arc A5437 (73.9284, 18.408) -> (73.8069, 18.7014) centre (73.8676, 18.5547) ccw
  arc A5438 (79.2554, 18.0447) -> (79.4799, 17.8201) centre (79.3676, 17.9324) ccw
  arc A5439 (73.5177, 27.2925) -> (73.2002, 27.2925) centre (73.359, 27.2925) ccw
  arc A5440 (72.2312, 25.4) -> (72.5487, 25.4) centre (72.3899, 25.4) ccw
  arc A5441 (71.8797, 26.7906) -> (71.8797, 26.4731) centre (71.8797, 26.6319) ccw
  line L1965 (72.8653, 17.9324) -> (71.314, 17.9324)
  arc A5442 (74.6442, 28.9826) -> (74.9617, 28.9826) centre (74.8029, 28.9826) ccw
  arc A5443 (80.4308, 18.408) -> (80.3093, 18.7014) centre (80.3701, 18.5547) ccw
  arc A5444 (79.6605, 18.4326) -> (79.782, 18.1393) centre (79.7212, 18.2859) ccw
  line L1966 (72.39, 24.1681) -> (72.9003, 24.1681)
  arc A5445 (71.314, 18.0911) -> (71.314, 17.7736) centre (71.314, 17.9323) ccw
  arc A5446 (69.9162, 19.5548) -> (69.6917, 19.3303) centre (69.804, 19.4426) ccw
  line L1967 (74.803, 29.4567) -> (74.93, 29.5837)
  arc A5447 (72.5487, 26.6319) -> (72.2312, 26.6319) centre (72.3899, 26.6319) ccw
  arc A5448 (71.4692, 21.9976) -> (71.7867, 21.9976) centre (71.6279, 21.9976) ccw
  arc A5449 (75.0423, 29.4714) -> (74.8177, 29.6959) centre (74.93, 29.5837) ccw
  line L1968 (74.93, 29.5837) -> (75.2, 29.3137)
  arc A5450 (72.39, 24.3269) -> (72.39, 24.0094) centre (72.39, 24.1682) ccw
  arc A5451 (71.7867, 24.4198) -> (71.4692, 24.4198) centre (71.6279, 24.4198) ccw
  line L1969 (71.314, 17.9324) -> (69.8039, 19.4425)
  arc A5452 (74.5699, 18.3959) -> (74.5699, 18.7134) centre (74.5699, 18.5547) ccw
  arc A5453 (75.158, 18.1393) -> (75.2795, 18.4326) centre (75.2188, 18.2859) ccw
  arc A5454 (73.7342, 24.7775) -> (73.5096, 25.002) centre (73.6219, 24.8897) ccw
  arc A5455 (71.4692, 26.3802) -> (71.7867, 26.3802) centre (71.6279, 26.3802) ccw
  line L1970 (74.803, 28.9826) -> (74.803, 29.4567)
  line L1971 (71.628, 26.3802) -> (71.628, 26.797)
  line L1972 (71.454, 21.5775) -> (71.628, 21.9976)
  line L1973 (75.2188, 18.2859) -> (74.5699, 18.5547)
  line L1974 (72.9003, 26.6319) -> (72.39, 26.6319)
  arc A5456 (79.3677, 17.7736) -> (79.3677, 18.0911) centre (79.3677, 17.9323) ccw
  arc A5457 (72.9003, 24.0094) -> (72.9003, 24.3269) centre (72.9003, 24.1682) ccw
  arc A5458 (71.2018, 17.8201) -> (71.4263, 18.0447) centre (71.3141, 17.9324) ccw
  arc A5459 (69.6917, 19.5548) -> (69.9162, 19.3303) centre (69.804, 19.4426) ccw
  line L1975 (72.39, 24.1681) -> (72.39, 25.4)
  line L1976 (70.0659, 20.1895) -> (71.454, 21.5775)
  line L1977 (71.8797, 26.6319) -> (71.628, 26.3802)
  arc A5460 (74.9497, 28.9219) -> (74.6563, 29.0434) centre (74.803, 28.9827) ccw
  line L1978 (79.7212, 18.2859) -> (79.3677, 17.9324)
  line L1979 (72.39, 26.6319) -> (72.39, 25.4)
  arc A5461 (72.753, 18.0447) -> (72.9775, 17.8201) centre (72.8653, 17.9324) ccw
  arc A5462 (70.1781, 19.5923) -> (69.9536, 19.8168) centre (70.0658, 19.7046) ccw
  arc A5463 (69.9536, 20.3017) -> (70.1781, 20.0772) centre (70.0659, 20.1895) ccw
  arc A5464 (71.5662, 21.4653) -> (71.3417, 21.6898) centre (71.454, 21.5776) ccw
  arc A5465 (70.2246, 20.1895) -> (69.9071, 20.1895) centre (70.0658, 20.1895) ccw
  arc A5466 (72.2313, 25.4) -> (72.5488, 25.4) centre (72.3901, 25.4) ccw
  arc A5467 (79.8335, 18.1737) -> (79.609, 18.3982) centre (79.7212, 18.2859) ccw
  arc A5468 (74.4823, 28.6233) -> (74.7757, 28.5018) centre (74.629, 28.5626) ccw
  line L1980 (73.6219, 25.4) -> (72.39, 25.4)
  arc A5469 (72.9003, 26.4731) -> (72.9003, 26.7906) centre (72.9003, 26.6319) ccw
  arc A5470 (73.4712, 27.1803) -> (73.2467, 27.4048) centre (73.359, 27.2926) ccw
  arc A5471 (73.0982, 26.8243) -> (72.9767, 27.1177) centre (73.0375, 26.971) ccw
  arc A5472 (73.8677, 18.7134) -> (73.8677, 18.3959) centre (73.8677, 18.5547) ccw
  arc A5473 (75.4601, 17.8201) -> (75.6846, 18.0447) centre (75.5724, 17.9324) ccw
  arc A5474 (80.3701, 18.7134) -> (80.3701, 18.3959) centre (80.3701, 18.5547) ccw
  arc A5475 (75.5723, 18.0911) -> (75.5723, 17.7736) centre (75.5723, 17.9323) ccw
  line L1981 (72.39, 25.4) -> (73.6219, 25.4)
  line L1982 (75.5723, 17.9324) -> (75.2188, 18.2859)
  line L1983 (77.47, 29.5837) -> (77.74, 29.3137)
  line L1984 (77.74, 29.3137) -> (78.3889, 29.0449)
  line L1985 (80.2955, 29.6574) -> (80.4879, 29.5176)
  arc A5476 (80.1832, 29.5452) -> (80.4077, 29.7697) centre (80.2955, 29.6575) ccw
  arc A5477 (78.3281, 28.8982) -> (78.4496, 29.1916) centre (78.3889, 29.0449) ccw
  line L1986 (81.28, 29.2989) -> (81.28, 31.75)
  arc A5478 (72.39, 26.4731) -> (72.39, 26.7906) centre (72.39, 26.6319) ccw
  arc A5479 (73.4631, 24.8897) -> (73.7806, 24.8897) centre (73.6218, 24.8897) ccw
  line L1987 (75.8489, 29.0449) -> (76.5511, 29.0449)
  arc A5480 (72.39, 25.5588) -> (72.39, 25.2413) centre (72.39, 25.4001) ccw
  arc A5481 (73.4631, 25.4) -> (73.7806, 25.4) centre (73.6218, 25.4) ccw
  arc A5482 (72.39, 26.7906) -> (72.39, 26.4731) centre (72.39, 26.6319) ccw
  arc A5483 (73.6219, 25.2413) -> (73.6219, 25.5588) centre (73.6219, 25.4001) ccw
  arc A5484 (77.6278, 29.2014) -> (77.8523, 29.4259) centre (77.74, 29.3136) ccw
  arc A5485 (71.628, 26.9558) -> (71.628, 26.6382) centre (71.628, 26.797) ccw
  line L1988 (74.629, 28.5625) -> (74.803, 28.9826)
  line L1989 (76.5511, 29.0449) -> (77.2, 29.3137)
  arc A5486 (77.8008, 29.4603) -> (77.6793, 29.167) centre (77.74, 29.3137) ccw
  arc A5487 (79.0304, 29.1916) -> (79.1519, 28.8982) centre (79.0911, 29.0449) ccw
  arc A5488 (73.6219, 25.2412) -> (73.6219, 25.5587) centre (73.6219, 25.4) ccw
  arc A5489 (81.28, 31.9087) -> (81.28, 31.5912) centre (81.28, 31.75) ccw
  arc A5490 (81.1362, 29.1421) -> (81.1859, 29.4557) centre (81.1611, 29.2989) ccw
  arc A5491 (72.788, 24.2804) -> (73.0125, 24.0558) centre (72.9003, 24.1681) ccw
  arc A5492 (72.39, 25.5587) -> (72.39, 25.2412) centre (72.39, 25.4) ccw
  arc A5493 (72.39, 25.5588) -> (72.39, 25.2413) centre (72.39, 25.4001) ccw
  arc A5494 (71.7867, 26.797) -> (71.4692, 26.797) centre (71.6279, 26.797) ccw
  arc A5495 (73.2002, 27.2925) -> (73.5177, 27.2925) centre (73.359, 27.2925) ccw
  line L1990 (79.0911, 29.0449) -> (79.74, 29.3137)
  arc A5496 (78.3889, 29.2037) -> (78.3889, 28.8862) centre (78.3889, 29.045) ccw
  arc A5497 (81.1212, 29.2989) -> (81.4387, 29.2989) centre (81.2799, 29.2989) ccw
  arc A5498 (75.0423, 29.6959) -> (74.8177, 29.4714) centre (74.93, 29.5836) ccw
  line L1991 (81.28, 31.75) -> (81.28, 29.2989)
  arc A5499 (81.4388, 31.75) -> (81.1213, 31.75) centre (81.2801, 31.75) ccw
  arc A5500 (75.7881, 28.8982) -> (75.9096, 29.1916) centre (75.8488, 29.0449) ccw
  arc A5501 (74.7412, 28.4503) -> (74.5167, 28.6748) centre (74.629, 28.5626) ccw
  arc A5502 (74.6907, 29.5689) -> (74.9153, 29.3444) centre (74.803, 29.4566) ccw
  line L1992 (72.39, 25.4) -> (72.39, 26.6319)
  arc A5503 (81.1611, 29.4577) -> (81.1611, 29.1401) centre (81.1611, 29.2989) ccw
  arc A5504 (71.992, 26.5196) -> (71.7675, 26.7441) centre (71.8798, 26.6319) ccw
  arc A5505 (71.5157, 26.4924) -> (71.7403, 26.2679) centre (71.628, 26.3802) ccw
  arc A5506 (73.5096, 25.798) -> (73.7342, 26.0225) centre (73.6219, 25.9103) ccw
  line L1993 (72.9003, 24.1681) -> (73.6219, 24.8897)
  arc A5507 (72.5488, 26.6319) -> (72.2313, 26.6319) centre (72.3901, 26.6319) ccw
  arc A5508 (81.28, 31.5912) -> (81.28, 31.9087) centre (81.28, 31.75) ccw
  arc A5509 (73.2467, 27.4048) -> (73.4712, 27.1803) centre (73.359, 27.2926) ccw
  line L1994 (73.359, 27.2925) -> (74.629, 28.5625)
  arc A5510 (72.6174, 26.6382) -> (72.6174, 26.9558) centre (72.6174, 26.797) ccw
  line L1995 (73.6219, 25.4) -> (73.6219, 25.9103)
  arc A5511 (72.5566, 26.9437) -> (72.6781, 26.6503) centre (72.6174, 26.797) ccw
  arc A5512 (72.9252, 27.0833) -> (73.1497, 26.8588) centre (73.0375, 26.9711) ccw
  line L1996 (80.9261, 29.3361) -> (81.1611, 29.2989)
  line L1997 (73.0375, 26.971) -> (73.359, 27.2925)
  line L1998 (71.628, 26.797) -> (72.6174, 26.797)
  arc A5513 (73.7806, 25.4) -> (73.4631, 25.4) centre (73.6218, 25.4) ccw
  line L1999 (73.6219, 24.8897) -> (73.6219, 25.4)
  arc A5514 (72.5488, 25.4) -> (72.2313, 25.4) centre (72.3901, 25.4) ccw
  arc A5515 (72.2313, 25.4) -> (72.5488, 25.4) centre (72.3901, 25.4) ccw
  arc A5516 (80.3019, 29.8755) -> (80.0773, 29.651) centre (80.1896, 29.7633) ccw
  line L2000 (80.1896, 29.7633) -> (80.2955, 29.6574)
  arc A5517 (80.3888, 29.7859) -> (80.2021, 29.529) centre (80.2954, 29.6575) ccw
  line L2001 (73.6219, 25.9103) -> (72.9003, 26.6319)
  line L2002 (72.6174, 26.797) -> (73.0375, 26.971)
  line L2003 (72.39, 26.6319) -> (71.8797, 26.6319)
  arc A5518 (77.5823, 29.6959) -> (77.3577, 29.4714) centre (77.47, 29.5837) ccw
  arc A5519 (82.9051, 30.4072) -> (82.6031, 30.5054) centre (82.7541, 30.4563) ccw
  line L2004 (81.28, 29.2989) -> (81.3989, 29.2989)
  arc A5520 (81.1213, 29.2989) -> (81.4388, 29.2989) centre (81.2801, 29.2989) ccw
  arc A5521 (81.9092, 29.2586) -> (81.8111, 29.5606) centre (81.8602, 29.4096) ccw
  line L2005 (81.3989, 29.2989) -> (81.6339, 29.3361)
  arc A5522 (81.3989, 29.1401) -> (81.3989, 29.4577) centre (81.3989, 29.2989) ccw
  arc A5523 (79.6277, 29.4259) -> (79.8522, 29.2014) centre (79.74, 29.3137) ccw
  line L2006 (81.1611, 29.2989) -> (81.28, 29.2989)
  arc A5524 (80.6278, 29.2682) -> (80.7719, 29.5511) centre (80.6998, 29.4097) ccw
  arc A5525 (75.2608, 29.4603) -> (75.1393, 29.167) centre (75.2001, 29.3137) ccw
  arc A5526 (81.4388, 31.75) -> (81.1213, 31.75) centre (81.2801, 31.75) ccw
  arc A5527 (82.4441, 33.3886) -> (82.701, 33.5752) centre (82.5726, 33.4819) ccw
  arc A5528 (81.6091, 34.0071) -> (81.6587, 34.3207) centre (81.6339, 34.1639) ccw
  line L2007 (82.7541, 33.0437) -> (82.6806, 33.2699)
  arc A5529 (80.877, 29.1851) -> (80.9752, 29.4871) centre (80.9261, 29.3361) ccw
  arc A5530 (77.2607, 29.167) -> (77.1392, 29.4603) centre (77.2, 29.3137) ccw
  arc A5531 (81.4387, 31.75) -> (81.1212, 31.75) centre (81.2799, 31.75) ccw
  arc A5532 (81.28, 34.3598) -> (81.28, 34.0423) centre (81.28, 34.2011) ccw
  arc A5533 (82.95, 32.8087) -> (82.6325, 32.8087) centre (82.7913, 32.8087) ccw
  arc A5534 (81.7881, 29.5511) -> (81.9322, 29.2682) centre (81.8602, 29.4096) ccw
  arc A5535 (82.4311, 30.0902) -> (82.714, 29.946) centre (82.5725, 30.0181) ccw
  arc A5536 (80.3019, 29.651) -> (80.0773, 29.8755) centre (80.1896, 29.7633) ccw
  arc A5537 (82.545, 29.7134) -> (82.3205, 29.9379) centre (82.4327, 29.8257) ccw
  line L2008 (81.6339, 34.1639) -> (81.3989, 34.2011)
  arc A5538 (79.8007, 29.167) -> (79.6792, 29.4603) centre (79.74, 29.3137) ccw
  arc A5539 (76.5511, 28.8862) -> (76.5511, 29.2037) centre (76.5511, 29.045) ccw
  arc A5540 (81.3741, 29.4557) -> (81.4238, 29.1421) centre (81.399, 29.2989) ccw
  arc A5541 (80.56, 29.6591) -> (80.4158, 29.3762) centre (80.4879, 29.5177) ccw
  line L2009 (82.4328, 33.6743) -> (82.2645, 33.8426)
  line L2010 (82.7913, 31.75) -> (81.28, 31.75)
  line L2011 (82.7913, 32.8087) -> (82.7541, 33.0437)
  arc A5542 (81.28, 31.9088) -> (81.28, 31.5913) centre (81.28, 31.7501) ccw
  line L2012 (82.6806, 33.2699) -> (82.5726, 33.4819)
  arc A5543 (77.0877, 29.4259) -> (77.3122, 29.2014) centre (77.2, 29.3136) ccw
  line L2013 (79.74, 29.3137) -> (80.1896, 29.7633)
  arc A5544 (81.28, 29.1401) -> (81.28, 29.4577) centre (81.28, 29.2989) ccw
  arc A5545 (80.7489, 29.5606) -> (80.6508, 29.2586) centre (80.6999, 29.4096) ccw
  line L2014 (75.2, 29.3137) -> (75.8489, 29.0449)
  arc A5546 (75.8489, 29.2037) -> (75.8489, 28.8862) centre (75.8489, 29.045) ccw
  arc A5547 (81.4238, 34.3579) -> (81.3741, 34.0443) centre (81.399, 34.2011) ccw
  line L2015 (80.4879, 29.5176) -> (80.6999, 29.4096)
  arc A5548 (76.4904, 29.1916) -> (76.6119, 28.8982) centre (76.5512, 29.0449) ccw
  line L2016 (82.2645, 29.6574) -> (82.4328, 29.8257)
  line L2017 (81.3989, 34.2011) -> (81.28, 34.2011)
  arc A5549 (82.5612, 33.7677) -> (82.3043, 33.581) centre (82.4327, 33.6744) ccw
  arc A5550 (82.714, 33.554) -> (82.4311, 33.4098) centre (82.5726, 33.4819) ccw
  line L2018 (80.6999, 29.4096) -> (80.9261, 29.3361)
  arc A5551 (80.9509, 29.4929) -> (80.9013, 29.1793) centre (80.9261, 29.3361) ccw
  line L2019 (82.0721, 33.9824) -> (81.8601, 34.0904)
  arc A5552 (79.0911, 28.8862) -> (79.0911, 29.2037) centre (79.0911, 29.045) ccw
  line L2020 (81.8601, 29.4096) -> (82.0721, 29.5176)
  arc A5553 (77.5823, 29.4714) -> (77.3577, 29.6959) centre (77.47, 29.5837) ccw
  arc A5554 (81.28, 29.4577) -> (81.28, 29.1401) centre (81.28, 29.2989) ccw